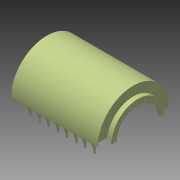
# Autodesk Inventor part: 主动轮护盖
Saved by Autodesk Inventor 2015 (Build 190159000, 159)
## iProperties
Created: 2017-05-11
Part Number: 主动轮护盖
Material: 常规
Document SubType Name: Modeling
Designer: Administrator
Density: 1 g/cm^3
Appearance: 铬酸锌 2
Author: Administrator
Autodesk Inventor part; units mm, degrees
ref_plane "YZ Plane" through (0, 0, 0) normal (1, 0, 0) x (0, 1, 0)
ref_plane "XZ Plane" through (0, 0, 0) normal (0, 1, 0) x (-1, 0, 0)
ref_plane "XY Plane" through (0, 0, 0) normal (0, 0, 1) x (1, 0, 0)
sketch "草图1" plane through (0, 0, 0) normal (0, 0, 1) x (1, 0, 0)
  circle A0 centre (0, 0) radius 141.3842
  line L0 (50, 166.3842) -> (50, 141.3842)
  line L1 (50, 141.3842) -> (-50, 141.3842)
  line L2 (-50, 141.3842) -> (-50, 166.3842)
  line L3 (-57.3473, 163.9969) -> (-42.6527, 143.7715)
  line L4 (-42.6527, 143.7715) -> (-123.5544, 84.9929)
  line L5 (-123.5544, 84.9929) -> (-138.249, 105.2184)
  line L6 (-142.7899, 98.9684) -> (-119.0135, 91.2429)
  line L7 (-119.0135, 91.2429) -> (-149.9152, -3.8627)
  line L8 (-149.9152, -3.8627) -> (-173.6916, 3.8627)
  line L9 (-173.6916, -3.8627) -> (-149.9152, 3.8627)
  line L10 (-149.9152, 3.8627) -> (-119.0135, -91.2429)
  line L11 (-119.0135, -91.2429) -> (-142.7899, -98.9684)
  line L12 (-138.249, -105.2184) -> (-123.5544, -84.9929)
  line L13 (-123.5544, -84.9929) -> (-42.6527, -143.7715)
  line L14 (-42.6527, -143.7715) -> (-57.3473, -163.9969)
  line L15 (-50, -166.3842) -> (-50, -141.3842)
  line L16 (-50, -141.3842) -> (50, -141.3842)
  line L17 (50, -141.3842) -> (50, -166.3842)
  line L18 (57.3473, -163.9969) -> (42.6527, -143.7715)
  line L19 (42.6527, -143.7715) -> (123.5544, -84.9929)
  line L20 (123.5544, -84.9929) -> (138.249, -105.2184)
  line L21 (142.7899, -98.9684) -> (119.0135, -91.2429)
  line L22 (119.0135, -91.2429) -> (149.9152, 3.8627)
  line L23 (149.9152, 3.8627) -> (173.6916, -3.8627)
  line L24 (173.6916, 3.8627) -> (149.9152, -3.8627)
  line L25 (149.9152, -3.8627) -> (119.0135, 91.2429)
  line L26 (119.0135, 91.2429) -> (142.7899, 98.9684)
  line L27 (138.249, 105.2184) -> (123.5544, 84.9929)
  line L28 (123.5544, 84.9929) -> (42.6527, 143.7715)
  line L29 (42.6527, 143.7715) -> (57.3473, 163.9969)
  line L30 (11.529, 166.3842) -> (50, 166.3842)
  line L31 (-315, 173.8842) -> (-280, 173.8842)
  line L32 (-280, 173.8842) -> (-280, 168.8842)
  line L33 (-280, 168.8842) -> (-315, 168.8842)
  line L34 (-315, 168.8842) -> (-315, 173.8842)
  line L35 (-315, 168.8842) -> (-310, 168.8842)
  line L36 (-310, 168.8842) -> (-310, 138.8842)
  line L37 (-310, 138.8842) -> (-315, 138.8842)
  line L38 (-315, 138.8842) -> (-315, 168.8842)
  line L39 (-280, 173.8842) -> (-285, 173.8842)
  line L40 (-285, 173.8842) -> (-285, 235)
  line L41 (-285, 235) -> (-280, 235)
  line L42 (-280, 235) -> (-280, 173.8842)
  line L43 (-280, 235) -> (280, 235)
  line L44 (280, 235) -> (280, 230)
  line L45 (280, 230) -> (-280, 230)
  line L46 (-280, 230) -> (-280, 235)
  line L47 (280, 235) -> (285, 235)
  line L48 (285, 235) -> (285, 173.8842)
  line L49 (285, 173.8842) -> (280, 173.8842)
  line L50 (280, 173.8842) -> (280, 235)
  line L51 (280, 173.8842) -> (315, 173.8842)
  line L52 (315, 173.8842) -> (315, 168.8842)
  line L53 (315, 168.8842) -> (280, 168.8842)
  line L54 (280, 168.8842) -> (280, 173.8842)
  line L55 (315, 168.8842) -> (310, 168.8842)
  line L56 (310, 168.8842) -> (310, 138.8842)
  line L57 (310, 138.8842) -> (315, 138.8842)
  line L58 (315, 138.8842) -> (315, 168.8842)
  line L59 (-213, 230) -> (-210, 230)
  line L60 (-210, 230) -> (-210, 175)
  line L61 (-210, 175) -> (-213, 175)
  line L62 (-213, 175) -> (-213, 230)
  line L63 (-150, 230) -> (-147, 230)
  line L64 (-147, 230) -> (-147, 175)
  line L65 (-147, 175) -> (-150, 175)
  line L66 (-150, 175) -> (-150, 230)
  line L67 (-93, 230) -> (-90, 230)
  line L68 (-90, 230) -> (-90, 175)
  line L69 (-90, 175) -> (-93, 175)
  line L70 (-93, 175) -> (-93, 230)
  line L71 (-30, 230) -> (-27, 230)
  line L72 (-27, 230) -> (-27, 175)
  line L73 (-27, 175) -> (-30, 175)
  line L74 (-30, 175) -> (-30, 230)
  line L75 (27, 230) -> (30, 230)
  line L76 (30, 230) -> (30, 175)
  line L77 (30, 175) -> (27, 175)
  line L78 (27, 175) -> (27, 230)
  line L79 (90, 230) -> (93, 230)
  line L80 (93, 230) -> (93, 175)
  line L81 (93, 175) -> (90, 175)
  line L82 (90, 175) -> (90, 230)
  line L83 (147, 230) -> (150, 230)
  line L84 (150, 230) -> (150, 175)
  line L85 (150, 175) -> (147, 175)
  line L86 (147, 175) -> (147, 230)
  line L87 (210, 230) -> (213, 230)
  line L88 (213, 230) -> (213, 175)
  line L89 (213, 175) -> (210, 175)
  line L90 (210, 175) -> (210, 230)
  line L91 (-441, 0) -> (441, 0) projected
  point P0 (0, 141.3842)
  point P1 (-83.1035, 114.3822)
  point P2 (-134.4643, 43.6901)
  point P3 (-134.4643, -43.6901)
  point P4 (-83.1035, -114.3822)
  point P5 (0, -141.3842)
  point P6 (83.1035, -114.3822)
  point P7 (134.4643, -43.6901)
  point P8 (134.4643, 43.6901)
  point P9 (83.1035, 114.3822)
  point P10 (50, 153.8842)
  dimension "d0" = 100
  dimension "d1" = 25
  dimension "d4" = 360
  dimension "d6" = 35
  dimension "d7" = 2.5
  dimension "d8" = 5
  dimension "d9" = 280
  dimension "d10" = 5
  dimension "d11" = 30
  dimension "d12" = 5
  dimension "d13" = 235
  dimension "d14" = 560
  dimension "d15" = 5
  dimension "d16" = 5
  dimension "d17" = 35
  dimension "d18" = 5
  dimension "d19" = 5
  dimension "d20" = 3
  dimension "d21" = 210
  dimension "d22" = 3
  dimension "d23" = 60
  dimension "d24" = 55
  dimension "d25" = 3
  dimension "d26" = 3
  dimension "d27" = 3
  dimension "d28" = 3
  dimension "d29" = 3
  dimension "d30" = 3
  dimension "d31" = 120
  dimension "d32" = 60
  dimension "d33" = 120
  dimension "d34" = 60
  dimension "d35" = 120
  dimension "d36" = 60
  constraints: 180 end point, 38 parallel, 18 horizontal, 16 perpendicular, 3 midpoint, 2 point on line, 1 coincident, 1 collinear, 1 vertical alignment, 94 other
  measures "d0" distance of L0.end L1.end
  measures "d1" distance of L0.start L0.end
  measures "d6" distance of L32.end L33.end
  measures "d7" distance between parallel lines of L33 L30
  measures "d8" distance of L33.end L31.start
  measures "d9" distance from line of point (0, 0) L32
  measures "d10" distance of L36.end L37.end
  measures "d11" distance of L37.end L33.end
  measures "d12" distance of L40.end L41.end
  measures "d13" distance from line of point (0, 0) L41
  measures "d14" distance of L44.end L46.start
  measures "d16" distance of L48.end L49.end
  measures "d17" distance of L52.end L53.end
  measures "d18" distance between parallel lines of L53 L51
  measures "d19" distance of L57.end L56.end
  measures "d20" distance of L60.end L61.end
  measures "d21" distance from line of point (0, 0) L60
  measures "d22" distance of L64.end L65.end
  measures "d23" distance between parallel lines of L60 L66
  measures "d24" distance of L61.end L59.start
  measures "d25" distance of L68.end L69.end
  measures "d26" distance of L72.end L73.end
  measures "d27" distance of L76.end L77.end
  measures "d28" distance of L80.end L81.end
  measures "d29" distance of L84.end L85.end
  measures "d30" distance of L88.end L89.end
  measures "d31" distance between parallel lines of L60 L68
  measures "d32" distance between parallel lines of L74 L68
  measures "d33" distance between parallel lines of L76 L68
  measures "d34" distance between parallel lines of L82 L76
  measures "d35" distance between parallel lines of L84 L76
  measures "d36" distance between parallel lines of L90 L84
revolve "旋转1" add sketch "草图1" angle 180 about axis through (-10, 0, 0) along (1, 0, 0) contours L31 L32 L33 L34 | L40 L41 L42 L31 | L33 L36 L37 L38 | L42 L43 L44 L45 | L45 L60 L61 L62 | L47 L48 L49 L50 L44 | L45 L64 L65 L66 | L88 L89 L90 L45 | L49 L51 L52 L53 L54 | L45 L68 L69 L70 | L84 L85 L86 L45 | L53 L58 L57 L56 | L45 L72 L73 L74 | L80 L81 L82 L45 | L45 L76 L77 L78
sketch "草图2" plane through (-315, 138.8842, 0) normal (-1, 0, 0) x (0, 0, 1)
  circle A0 centre (10, 13.7887) radius 2.5
  arc A1 (27.2318, 11.6729) -> (10, 13.7887) centre (0, -138.8842) ccw
  arc A2 (0, -277.7684) -> (0, 0) centre (0, -138.8842) ccw projected
  line L0 (0, 35) -> (0, 0) projected
  line L1 (10, 13.7887) -> (0, -138.8842)
  point P0 (0, -138.8842)
  dimension "d38" = 5
  dimension "d39" = 153
  dimension "d40" = 10
  constraints: 2 centre point, 2 end point, 2 point on circle, 1 concentric
  measures "d38" diameter of A0
  measures "d39" radius of A1
  measures "d40" distance from line of L1.start L0
extrude "拉伸1" cut sketch "草图2" against normal through all
pattern_circular "环形阵列1" count 6 over 172.5 about axis through (-312.5, 0, 0) along (1, 0, 0) of "拉伸1"
sketch "草图3" plane through (285, -235, 0) normal (0, 0, -1) x (-1, 0, 0)
  line L0 (72, 60) -> (75, 60)
  line L1 (75, 60) -> (75, 5)
  line L2 (75, 5) -> (72, 5)
  line L3 (72, 5) -> (72, 60)
  line L4 (135, 60) -> (138, 60)
  line L5 (138, 60) -> (138, 5)
  line L6 (138, 5) -> (135, 5)
  line L7 (135, 5) -> (135, 60)
  line L8 (192, 60) -> (195, 60)
  line L9 (195, 60) -> (195, 5)
  line L10 (195, 5) -> (192, 5)
  line L11 (192, 5) -> (192, 60)
  line L12 (255, 60) -> (258, 60)
  line L13 (258, 60) -> (258, 5)
  line L14 (258, 5) -> (255, 5)
  line L15 (255, 5) -> (255, 60)
  line L16 (312, 60) -> (315, 60)
  line L17 (315, 60) -> (315, 5)
  line L18 (315, 5) -> (312, 5)
  line L19 (312, 5) -> (312, 60)
  line L20 (375, 60) -> (378, 60)
  line L21 (378, 60) -> (378, 5)
  line L22 (378, 5) -> (375, 5)
  line L23 (375, 5) -> (375, 60)
  line L24 (432, 60) -> (435, 60)
  line L25 (435, 60) -> (435, 5)
  line L26 (435, 5) -> (432, 5)
  line L27 (432, 5) -> (432, 60)
  line L28 (495, 60) -> (498, 60)
  line L29 (498, 60) -> (498, 5)
  line L30 (498, 5) -> (495, 5)
  line L31 (495, 5) -> (495, 60)
  line L32 (565, 5) -> (498, 5) projected
  line L33 (498, 5) -> (498, 60) projected
  line L34 (135, 60) -> (135, 5) projected
  point P0 (285, 235)
  constraints: 64 end point, 16 parallel, 8 horizontal, 8 perpendicular, 3 collinear, 1 point on line
extrude "拉伸2" add sketch "草图3" along normal blind 100
sketch "草图4" plane through (213, 175, 0) normal (1, 0, 0) x (0, 0, -1)
  line L0 (100, -405) -> (100, -350) projected
  arc A0 (100, -360) -> (0, -405) centre (100, -493.6111) ccw
  line L1 (0, -405) -> (100, -405)
  line L2 (0, -410) -> (0, -348.8842) projected
  line L3 (100, -360) -> (100, -405)
  point P0 (0, -175)
  dimension "d48" = 10
  constraints: 4 end point, 2 point on circle, 1 centre point, 1 collinear, 1 line through centre, 1 perpendicular, 1 point on line
  measures "d48" distance of L0.end L3.start
extrude "拉伸3" cut sketch "草图4" against normal up to surface (426 mm away)
sketch "草图5" plane through (213, 175, 0) normal (1, 0, 0) x (0, 0, -1)
  circle A0 centre (94.9541, -355.0459) radius 5.0459
  line L0 (0, -350) -> (100, -350) projected
  line L1 (100, -350) -> (100, -360) projected
  arc A1 (100, -360) -> (0, -405) centre (100, -493.6111) ccw projected
  line L2 (94.9541, -350) -> (100, -350)
  line L3 (100, -350.2573) -> (100, -360)
  arc A2 (100, -360) -> (95.1377, -360.0885) centre (100, -493.6111) ccw
  point P0 (0, -175)
  constraints: 5 point on circle, 4 end point, 4 tangent, 2 centre point, 2 collinear, 2 point on line, 1 concentric
extrude "拉伸4" cut sketch "草图5" against normal up to surface (426 mm away) contours L1 A1 A0 | A0 L0 L1
sketch "草图6" plane through (285, -235, 0) normal (0, 0, -1) x (-1, 0, 0)
  line L0 (595, 0) -> (565, 0)
  line L1 (565, 0) -> (565, 96.1158)
  line L2 (565, 96.1158) -> (595, 96.1158)
  line L3 (595, 96.1158) -> (595, 0)
  line L4 (595, 96.1158) -> (595, 66.1158) projected
  line L5 (565, 66.1158) -> (565, 5) projected
  line L6 (0, 0) -> (570, 0) projected
  line L7 (600, 96.1158) -> (595, 96.1158) projected
  line L8 (-25, 96.1158) -> (5, 96.1158)
  line L9 (5, 96.1158) -> (5, 0)
  line L10 (5, 0) -> (-25, 0)
  line L11 (-25, 0) -> (-25, 96.1158)
  line L12 (-25, 66.1158) -> (-25, 96.1158) projected
  line L13 (-25, 96.1158) -> (-30, 96.1158) projected
  line L14 (5, 5) -> (5, 66.1158) projected
  point P0 (285, 235)
  constraints: 16 end point, 8 collinear, 4 parallel, 2 horizontal, 2 perpendicular
extrude "拉伸5" cut sketch "草图6" against normal blind 25
